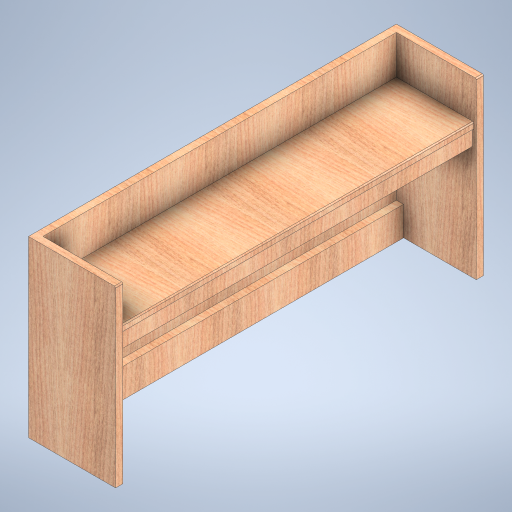
# Autodesk Inventor part: Shelf
Saved by Autodesk Inventor 2023 (Build 270158000, 158)
## iProperties
Created: 2022-09-18
Part Number: Shelf
Material: Wood (Birch)
Document SubType Name: Modeling
Designer: mliu-23
Density: 0.55 g/cm^3
Appearance: Birch - Natural Polished
Author: mliu-23
Autodesk Inventor part; units mm, degrees
ref_plane "YZ Plane" through (0, 0, 0) normal (1, 0, 0) x (0, 1, 0)
ref_plane "XZ Plane" through (0, 0, 0) normal (0, 1, 0) x (-1, 0, 0)
ref_plane "XY Plane" through (0, 0, 0) normal (0, 0, 1) x (1, 0, 0)
sketch "Sketch1" plane through (0, 0, 0) normal (0, 1, 0) x (-1, 0, 0)
  line L0 (0, 0) -> (228.6, 0)
  line L1 (228.6, 0) -> (228.6, -965.2)
  line L2 (228.6, -965.2) -> (0, -965.2)
  line L3 (0, -965.2) -> (0, 0)
  line L4 (0, -19.05) -> (209.55, -19.05)
  line L5 (209.55, -19.05) -> (209.55, -946.15)
  line L6 (209.55, -946.15) -> (0, -946.15)
  line L7 (0, -946.15) -> (0, -19.05)
  point P0 (0, -946.15)
  dimension "d0" = 228.6
  dimension "d1" = 965.2
  dimension "d2" = 19.05
  dimension "d3" = 19.05
  dimension "d4" = 19.05
  constraints: 16 end point, 4 parallel, 2 horizontal, 2 perpendicular, 1 point on line
  measures "d0" distance of L1.end L2.end
  measures "d1" distance of L0.end L1.end
  measures "d2" distance between parallel lines of L5 L1
  measures "d3" distance between parallel lines of L0 L4
  measures "d4" distance between parallel lines of L2 L6
extrude "Extrusion1" add sketch "Sketch1" along normal blind 457.2 contours L0 L1 L2 L3 L6 L5 L4
sketch "Sketch2" plane through (0, 0, 0) normal (0, -1, 0) x (1, 0, 0)
  line L0 (0, -19.05) -> (-209.55, -19.05) projected
  line L1 (-209.55, -19.05) -> (-209.55, -946.15) projected
  line L2 (-190.5, -19.05) -> (-209.55, -19.05)
  line L3 (-209.55, -19.05) -> (-209.55, -946.15)
  line L4 (-209.55, -946.15) -> (-190.5, -946.15)
  line L5 (-190.5, -946.15) -> (-190.5, -19.05)
  point P0 (0, 0)
  dimension "d7" = 19.05
  constraints: 8 end point, 2 parallel, 1 horizontal, 1 perpendicular, 1 point on line
  measures "d7" distance between parallel lines of L1 L5
extrude "Extrusion2" add sketch "Sketch2" against normal blind 76.2
sketch "Sketch3" plane through (-209.55, 457.2, -19.05) normal (1, 0, 0) x (0, 0, -1)
  line L0 (0, -381) -> (927.1, -381) projected
  line L1 (927.1, -381) -> (927.1, 0) projected
  line L2 (0, 0) -> (927.1, 0) projected
  line L3 (0, -381) -> (0, 0) projected
  line L4 (0, -457.2) -> (0, 0) projected
  line L5 (927.1, -457.2) -> (927.1, 0) projected
  line L6 (0, -101.6) -> (927.1, -101.6)
  line L7 (927.1, -101.6) -> (927.1, -120.65)
  line L8 (927.1, -120.65) -> (0, -120.65)
  line L9 (0, -120.65) -> (0, -101.6)
  point P0 (-19.05, -457.2)
  point P1 (0, -120.65)
  point P2 (927.1, -120.65)
  point P3 (927.1, -101.6)
  dimension "d10" = 19.05
  dimension "d11" = 101.6
  constraints: 8 end point, 2 parallel, 2 point on line, 1 horizontal, 1 perpendicular
  measures "d10" distance between parallel lines of L8 L6
  measures "d11" distance between parallel lines of L6 L2
extrude "Extrusion3" add sketch "Sketch3" along normal blind 203.2 contours L3 L6 L1 L8
sketch "Sketch4" plane through (-209.55, 336.55, -946.15) normal (0, -1, 0) x (1, 0, 0)
  line L0 (209.55, 927.1) -> (19.05, 927.1) projected
  line L1 (19.05, 0) -> (209.55, 0) projected
  line L2 (200.025, 927.1) -> (180.975, 927.1)
  line L3 (180.975, 927.1) -> (180.975, 0)
  line L4 (180.975, 0) -> (200.025, 0)
  line L5 (200.025, 0) -> (200.025, 927.1)
  line L6 (203.2, 927.1) -> (203.2, 0) projected
  point P0 (209.55, 946.15)
  point P1 (200.025, 0)
  dimension "d14" = 19.05
  dimension "d15" = 3.175
  constraints: 8 end point, 2 parallel, 2 point on line, 1 horizontal, 1 perpendicular
  measures "d14" distance between parallel lines of L3 L5
  measures "d15" distance between parallel lines of L6 L5
extrude "Extrusion4" add sketch "Sketch4" along normal blind 38.1 contours L5 L1 L3 L0
fillet "Fillet1" radius 3.175 4 edges at (-6.35, 355.6, -482.6) (-6.35, 336.55, -482.6) (0, 457.2, -9.525) (0, 457.2, -955.675)
body "Solid1"
